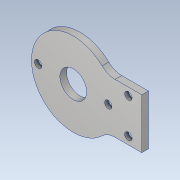
# Autodesk Inventor part: LowerArm_JointConnector_Prox_v2
Saved by Autodesk Inventor 2021.4 (Build 254397000, 397)
## iProperties
Created: 2020-04-27
Part Number: LowerArm_JointConnector_Prox_v2
Material: Aluminum 6061
Document SubType Name: Modeling
Designer: Alex
Density: 2.7 g/cm^3
Appearance: Aluminum - Flat
Mass: 2.95762 g
Surface Area: 14.0747 cm^2
Volume: 1.09541 cm^3
JointFixation_DiaOut: 25,000 mm
LowerArm_ShaftFixation_Width: 8,000 mm
ShaftFixation_Width: 15,000 mm
JointFixation_FixHole_Dia: 21,000 mm
LowerArm_ProximalJoint_BasePlate_Thickness: 2,000 mm
Author: Alex
Autodesk Inventor part; units mm, degrees
ref_plane "YZ Plane" through (0, 0, 0) normal (1, 0, 0) x (0, 1, 0)
ref_plane "XZ Plane" through (0, 0, 0) normal (0, 1, 0) x (-1, 0, 0)
ref_plane "XY Plane" through (0, 0, 0) normal (0, 0, 1) x (1, 0, 0)
sketch "Skizze1" plane through (0, 0, 0) normal (0, 0, 1) x (1, 0, 0)
  line L0 (0, 0) -> (20.5, 0) construction
  circle A0 centre (0, 0) radius 4
  arc A1 (8.6207, 9.0517) -> (12.5, 7.5) centre (12.5, 13.125) ccw
  arc A2 (12.5, -7.5) -> (8.6207, -9.0517) centre (12.5, -13.125) ccw
  line L1 (12.5, 7.5) -> (20.5, 7.5)
  line L2 (20.5, 7.5) -> (20.5, -7.5)
  line L3 (20.5, -7.5) -> (12.5, -7.5)
  line L4 (12.5, -7.5) -> (12.5, 7.5) construction
  circle A3 centre (0, 0) radius 10.5 construction
  line L5 (0, 0) -> (-10.5, 0) construction
  line L6 (16.5, 5.25) -> (16.5, -5.25) construction
  line L7 (16.5, 7.5) -> (16.5, -7.5) construction
  circle A4 centre (0, 0) radius 12.5
  point P0 (12.5, 0)
  point P1 (10.5, 0)
  point P2 (16.5, 0)
  dimension "d105" = 8
  dimension "d106" = 15
  dimension "LowerArm_ShaftFixation_Width" = 8
  dimension "d127" = 21
  dimension "d130" = 360
  dimension "d132" = 10.5
  dimension "d150" = 25
  constraints: 16 end point, 8 point on circle, 5 centre point, 5 midpoint, 4 coincident, 4 tangent, 3 point on line, 2 horizontal, 2 parallel, 1 collinear, 1 equal radius, 1 perpendicular, 1 vertical, 3 other
  measures "d105" diameter of A0
  measures "d106" distance between parallel lines of L3 L1
  measures "LowerArm_ShaftFixation_Width" distance between parallel lines of L2 L4
  measures "d127" diameter of A3
  measures "d132" distance of L6.start L6.end
  measures "d150" diameter of A4
extrude "Grundprofil" add sketch "Skizze1" along normal blind 2
hole "Hole10" at (10.5, 0, 0) at (-10.5, 0, 0) direction (0, 0, 1) diameter 2.2 depth 12 tip angle 118 countersink diameter 4.4 countersink angle 90 clearance for "Countersunk Flat Head Screw DIN EN ISO 2009" size "M2" standard "DIN"
hole "Hole11" at (16.5, 5.25, 0) at (16.5, -5.25, 0) direction (0, 0, 1) diameter 2.2 depth 3 tip angle 118 countersink diameter 4.4 countersink angle 90 clearance for "Countersunk Raised Head Screw ISO 2010/7047" size "M2" standard "ISO"
